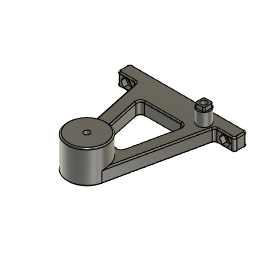
SpringFrameBack v2 (Autodesk Fusion 360 design; units mm, degrees)
Autodesk Fusion 360 part; units mm, degrees
sketch "bottom" plane through (0, 0, 0) normal (0, 0, 1) x (1, 0, 0)
  line L0 (-39.6542, 45.61) -> (46.3458, 45.61)
  line L1 (48.3458, 43.61) -> (48.3458, 37.61)
  line L2 (-41.6542, 37.61) -> (-41.6542, 43.61)
  circle A0 centre (25.8882, 34.76) radius 2.25
  arc A1 (46.3458, 35.61) -> (48.3458, 37.61) centre (46.3458, 37.61) ccw
  arc A2 (48.3458, 43.61) -> (46.3458, 45.61) centre (46.3458, 43.61) ccw
  arc A3 (-39.6542, 45.61) -> (-41.6542, 43.61) centre (-39.6542, 43.61) ccw
  arc A4 (-41.6542, 37.61) -> (-39.6542, 35.61) centre (-39.6542, 37.61) ccw
  line L3 (46.3458, 35.61) -> (34.9458, 35.61)
  line L4 (3.3458, -47.39) -> (3.3458, -32.39) construction
  circle A5 centre (3.3458, -32.39) radius 15
  line L5 (-26.299, 34.0309) -> (-11.3181, -35.5473)
  line L6 (32.9906, 34.0309) -> (18.0098, -35.5473)
  line L7 (46.3458, 35.61) -> (34.9458, 35.61)
  line L8 (-28.2542, 35.61) -> (-39.6542, 35.61)
  arc A6 (-26.299, 34.0309) -> (-28.2542, 35.61) centre (-28.2542, 33.61) ccw
  arc A7 (34.9458, 35.61) -> (32.9906, 34.0309) centre (34.9458, 33.61) ccw
  line L9 (3.3458, 45.61) -> (3.3458, 25.61) construction
  line L10 (3.3458, 25.61) -> (-10.5542, 25.61)
  line L11 (3.3458, 25.61) -> (17.2458, 25.61)
  line L12 (-13.487, 21.9785) -> (-5.9537, -13.0099)
  line L13 (20.1786, 21.9785) -> (12.6453, -13.0099)
  arc A8 (20.1786, 21.9785) -> (17.2458, 25.61) centre (17.2458, 22.61) ccw
  arc A9 (-10.5542, 25.61) -> (-13.487, 21.9785) centre (-10.5542, 22.61) ccw
  arc A10 (-5.9537, -13.0099) -> (-2.1113, -15.2372) centre (-3.0209, -12.3784) ccw
  arc A11 (8.803, -15.2372) -> (12.6453, -13.0099) centre (9.7125, -12.3784) ccw
  line L14 (3.3458, 45.61) -> (3.3458, 25.61) construction
  line L15 (3.3458, -14.39) -> (3.3458, -47.39) construction
  arc A12 (8.803, -15.2372) -> (-2.1113, -15.2372) centre (3.3458, -32.39) ccw
  arc A13 (34.9458, 35.61) -> (32.9906, 34.0309) centre (34.9458, 33.61) ccw
  circle A14 centre (3.3458, -32.39) radius 2.25
  circle A15 centre (25.8882, 34.76) radius 5
  line L16 (23.3882, 38.26) -> (28.3882, 38.26)
  line L17 (29.3882, 37.26) -> (29.3882, 32.26)
  line L18 (28.3882, 31.26) -> (23.3882, 31.26)
  line L19 (22.3882, 32.26) -> (22.3882, 37.26)
  line L20 (22.3882, 38.26) -> (29.3882, 31.26) construction
  line L21 (29.3882, 38.26) -> (22.3882, 31.26) construction
  arc A16 (23.3882, 38.26) -> (22.3882, 37.26) centre (23.3882, 37.26) ccw
  arc A17 (29.3882, 37.26) -> (28.3882, 38.26) centre (28.3882, 37.26) ccw
  arc A18 (22.3882, 32.26) -> (23.3882, 31.26) centre (23.3882, 32.26) ccw
  arc A19 (28.3882, 31.26) -> (29.3882, 32.26) centre (28.3882, 32.26) ccw
  point P0 (-41.6542, 45.61)
  point P1 (48.3458, 45.61)
  point P2 (-41.6542, 35.61)
  point P3 (25.8882, 34.76)
  dimension "d1" = 90
  dimension "d2" = 10
  dimension "d3" = 4.5
  dimension "d4" = 10.85
  dimension "d5" = 2
  dimension "d6" = 2
  dimension "d7" = 2
  dimension "d8" = 2
  dimension "d9" = 11.4
  dimension "d10" = 4
  dimension "d11" = 4
  dimension "d12" = 93
  dimension "d13" = 15
  dimension "d14" = 30
  dimension "d15" = 20
  dimension "d16" = 13.9
  dimension "d17" = 6
  dimension "d18" = 6
  dimension "d20" = 4.5
  dimension "d25" = 10
  dimension "d30" = 7
  dimension "d31" = 7
  dimension "d32" = 1
  dimension "d33" = 1
  dimension "d34" = 1
  dimension "d35" = 1
  constraint horizontal L0
  constraint vertical L1
  constraint horizontal L7
  constraint vertical L2
  constraint tangent L1 A1
  constraint tangent A1 L7
  constraint coincident P1 L0
  constraint coincident P1 L1
  constraint tangent L0 A2
  constraint tangent L1 A2
  constraint coincident P0 L0
  constraint coincident P0 L2
  constraint tangent L0 A3
  constraint tangent L2 A3
  constraint coincident P2 L7
  constraint coincident P2 L2
  constraint tangent A4 L7
  constraint tangent L2 A4
  constraint parallel L3 L7
  constraint tangent L3 A7
  constraint vertical L3.end A7.centre
  constraint vertical L14
  constraint midpoint L0 L9.start
  constraint symmetric A6 L14 A13
  constraint parallel L4 L14
  constraint coincident L4.end A5.centre
  constraint coincident A5 L5.end
  constraint symmetric L5.end L6.end L14
  constraint symmetric L5.start L6.start L14
  constraint collinear L7 L8
  constraint perpendicular L0 L9
  constraint perpendicular L9 L10
  constraint symmetric L10.end L11.end L14
  constraint tangent L10 A9
  constraint symmetric A8 A9 L14
  constraint tangent L12 A9
  constraint parallel L5 L12
  constraint tangent L12 A10
  constraint tangent A10 A12
  constraint symmetric A10 A11 L14
  constraint symmetric L12.end L13.end L14
  constraint coincident L15.start A12
  constraint collinear L14 L15
  constraint concentric A5 A12
  constraint concentric A12 A14
  constraint concentric A0 A15
  constraint horizontal L16
  constraint perpendicular L16 L17
  constraint parallel L16 L18
  constraint parallel L17 L19
  constraint coincident L20 P3
  constraint coincident L21 P3
  constraint coincident P3 A0.centre
  constraint coincident L20.start L16
  constraint coincident L20.start L19
  constraint tangent L16 A16
  constraint tangent L19 A16
  constraint coincident L21.start L16
  constraint coincident L21.start L17
  constraint tangent L16 A17
  constraint tangent L17 A17
  constraint coincident L21.end L19
  constraint coincident L21.end L18
  constraint tangent L19 A18
  constraint tangent L18 A18
  constraint coincident L20.end L17
  constraint coincident L20.end L18
  constraint tangent L17 A19
  constraint tangent L18 A19
  measures "d1" distance of P0 P1
  measures "d2" distance of P0 P2
  measures "d3" diameter of A0
  measures "d4" distance of L0 P3
  measures "d5" radius of A1
  measures "d6" radius of A2
  measures "d7" radius of A3
  measures "d8" radius of A4
  measures "d9" distance of A1.start L3.end
  measures "d10" diameter of A7
  measures "d11" diameter of A13
  measures "d12" distance of L9.start L4.start
  measures "d13" distance of L4.start L4.end
  measures "d14" diameter of A5
  measures "d15" distance of L9.start L9.end
  measures "d16" distance of L9.end L10.end
  measures "d17" diameter of A9
  measures "d18" diameter of A10
  measures "d20" diameter of A14
  measures "d25" diameter of A15
  measures "d30" distance of L20.end L21.end
  measures "d31" distance of L21.start L20.end
  measures "d32" radius of A16
  measures "d33" radius of A17
  measures "d34" radius of A18
  measures "d35" radius of A19
extrude "Extrude1" add sketch "bottom" along normal blind 10 contours L0 L1 L2 A1 A2 A3 A4 L3 A5 L5 L6 L7 L8 A6 A7 A13 | A5 | A15 | L16 L17 L18 L19 A16 A17 A18 A19
extrude "Extrude2" add sketch "bottom" along normal blind 25.5 contours A5
extrude "Extrude3" add sketch "bottom" along normal blind 20 contours A15 | L16 L17 L18 L19 A16 A17 A18 A19
extrude "Extrude4" add sketch "bottom" along normal blind 23 contours L16 L17 L18 L19 A16 A17 A18 A19
sketch "screw-hole" plane through (0, 35.61, 0) normal (0, -1, 0) x (1, 0, 0)
  line L0 (34.9458, 0) -> (46.3458, 0)
  line L1 (46.3458, 0) -> (46.3458, 10)
  line L2 (46.3458, 10) -> (34.9458, 10)
  line L3 (34.9458, 10) -> (34.9458, 0)
  line L4 (41.0825, 4.9942) -> (48.3325, 4.9942) construction
  line L5 (48.3325, 4.9942) -> (48.3325, -0.0058) construction
  line L6 (48.3325, -0.0058) -> (41.0825, -0.0058) construction
  line L7 (41.0825, -0.0058) -> (41.0825, 4.9942) construction
  circle A0 centre (41.0825, 4.9942) radius 2.25
  line L8 (45.2375, 4.9942) -> (43.16, 8.5925)
  line L9 (43.16, 8.5925) -> (39.005, 8.5925)
  line L10 (39.005, 8.5925) -> (36.9275, 4.9942)
  line L11 (36.9275, 4.9942) -> (39.005, 1.3959)
  line L12 (39.005, 1.3959) -> (43.16, 1.3959)
  line L13 (43.16, 1.3959) -> (45.2375, 4.9942)
  line L14 (3.3458, 0, -10) -> (3.3458, 0, 10)
  line L15 (-38.5459, 4.9942) -> (-36.4684, 8.5925)
  circle A1 centre (-34.3909, 4.9942) radius 2.25
  line L16 (-36.4684, 8.5925) -> (-32.3134, 8.5925)
  line L17 (-32.3134, 8.5925) -> (-30.2359, 4.9942)
  line L18 (-30.2359, 4.9942) -> (-32.3134, 1.3959)
  line L19 (-32.3134, 1.3959) -> (-36.4684, 1.3959)
  line L20 (-36.4684, 1.3959) -> (-38.5459, 4.9942)
  point P0 (41.0825, 4.9942)
  dimension "d38" = 7.25
  dimension "d39" = 5
  dimension "d40" = 4.5
  dimension "d41" = 4.155
  constraint horizontal L4
  constraint vertical L5
  constraint horizontal L6
  constraint vertical L7
  constraint coincident P0 L4.start
  constraint coincident L4 L8.start
  measures "d38" distance of P0 L4.end
  measures "d39" distance of P0 L6.end
  measures "d40" diameter of A0
  measures "d41" distance of L8.start P0
extrude "Extrude5" cut sketch "screw-hole" against normal blind 22 contours A0 | A1
extrude "Extrude6" cut sketch "screw-hole" against normal blind 3.5 contours L8 L9 L10 L11 L12 L13 | L15 L16 L17 L18 L19 L20
fillet "Fillet1" radius 1 13 edges at (25.5002, -0.7582, 10) (33.6892, 35.1659, 10) (40.6458, 35.61, 10) (47.76, 36.1957, 10) (48.3458, 40.61, 10) (47.76, 45.0242, 10) (3.3458, 45.61, 10) (-41.0684, 45.0242, 10) (-41.6542, 40.61, 10) (-41.0684, 36.1957, 10) (-33.9542, 35.61, 10) (-26.9976, 35.1659, 10) (-18.8086, -0.7582, 10)
fillet "Fillet1" radius 1 23 edges at (-10.6391, -37.8143, 25.5) (3.3458, -14.39, 10) (-4.5254, -14.9739, 10) (-9.7203, 4.4843, 10) (-12.8881, 24.4948, 10) (3.3458, 25.61, 10) (19.5797, 24.4949, 10) (16.4119, 4.4843, 10) (11.217, -14.9739, 10) (25.5002, -0.7582, 0) (33.6892, 35.1659, 0) (40.6458, 35.61, 0) (47.76, 36.1957, 0) (48.3458, 40.61, 0) (47.76, 45.0242, 0) (3.3458, 45.61, 0) (-41.0684, 45.0242, 0) (-41.6542, 40.61, 0) (-41.0684, 36.1957, 0) (-33.9542, 35.61, 0) (-26.9976, 35.1659, 0) (-18.8086, -0.7582, 0) (3.3458, -47.39, 0)
fillet "Fillet1" radius 1 8 edges at (16.4119, 4.4843, 0) (11.217, -14.9739, 0) (3.3458, -14.39, 0) (-4.5254, -14.9739, 0) (-9.7203, 4.4843, 0) (-12.8881, 24.4948, 0) (3.3458, 25.61, 0) (19.5797, 24.4949, 0)
equation "d4 = 8.60 mm + 2.25 mm"
equation "d16 = ( 27.80 / 2 ) * 1 mm"
equation "d41 = ( 8.31 / 2 ) * 1 mm"
named bodies: "SpringFrameBack"
